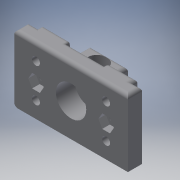
# Autodesk Inventor part: Upper_bearing_support_inside
Saved by Autodesk Inventor 2019.3 (Build 233278000, 278)
## iProperties
Created: 2020-09-08
Part Number: Upper_bearing_support_inside
Material: Generisch
Document SubType Name: Modeling
Designer: Nicolas Frick
Density: 1 g/cm^3
Appearance: Vorgabe
Author: Nicolas Frick
Autodesk Inventor part; units mm, degrees
ref_plane "YZ Plane" through (0, 0, 0) normal (1, 0, 0) x (0, 1, 0)
ref_plane "XZ Plane" through (0, 0, 0) normal (0, 1, 0) x (-1, 0, 0)
ref_plane "XY Plane" through (0, 0, 0) normal (0, 0, 1) x (1, 0, 0)
sketch "Skizze1" plane through (0, 0, 0) normal (0, 0, 1) x (1, 0, 0)
  line L0 (0, 81) -> (-70, 81) construction
  line L1 (-70, 0) -> (-70, 81) construction
  line L2 (-55.2549, 0) -> (-70, 0) construction
  line L3 (-55.2549, 0) -> (-55.2549, 27) construction
  line L4 (-55.2549, 27) -> (-15.0049, 27) construction
  line L5 (-15.0049, 27) -> (-15.0049, 0) construction
  line L6 (0, 0) -> (-15.0049, 0) construction
  line L7 (0, 0) -> (0, 81) construction
  line L8 (-35.1299, 27) -> (-35.1299, 54) construction
  line L9 (-65.1299, 36.5) -> (-5.1299, 36.5)
  line L10 (-5.1299, 36.5) -> (-5.1299, 71.5)
  line L11 (-5.1299, 71.5) -> (-65.1299, 71.5)
  line L12 (-65.1299, 71.5) -> (-65.1299, 36.5)
  line L13 (-65.1299, 36.5) -> (-5.1299, 71.5) construction
  line L14 (-5.1299, 36.5) -> (-65.1299, 71.5) construction
  circle A0 centre (-35.1299, 54) radius 8
  dimension "d0" = 27
  dimension "d1" = 60
  dimension "d2" = 35
  dimension "d3" = 16
  constraints: 14 end point, 3 midpoint, 2 parallel, 1 centre point, 1 coincident, 1 horizontal, 1 perpendicular, 1 vertical
  measures "d0" distance of L8.start L8.end
  measures "d1" distance of L11.end L10.end
  measures "d2" distance of L10.end L9.end
  measures "d3" diameter of A0
extrude "Extrusion1" add sketch "Skizze1" along normal blind 10
sketch "Skizze2" plane through (-65.1299, 71.5, 0) normal (0, 1, 0) x (1, 0, 0)
  line L0 (0, 0) -> (60, 0) construction
  line L1 (60, 0) -> (40, 0) construction
  line L2 (0, 0) -> (0, -10) construction
  line L3 (40, 0) -> (20, 0)
  line L4 (20, 0) -> (20, 10)
  line L5 (20, 10) -> (40, 10)
  line L6 (40, 10) -> (40, 0)
  circle A0 centre (30, 3.7987) radius 3.15
  point P0 (65.1299, 0)
  dimension "d6" = 20
  dimension "d7" = 20
  dimension "d8" = 10
  dimension "d9" = 6.3
  constraints: 10 end point, 2 parallel, 2 perpendicular, 1 centre point, 1 horizontal
  measures "d6" distance of L0.end L1.end
  measures "d7" distance of L4.end L5.end
  measures "d8" distance of L3.end L4.end
  measures "d9" diameter of A0
extrude "Extrusion2" add sketch "Skizze2" against normal up to surface (35 mm away)
sketch "Skizze3" plane through (-65.1299, 36.5, 10) normal (0, -1, 0) x (1, 0, 0)
  circle A0 centre (30, -13.7987) radius 3.15 construction
  line L0 (56.6201, -20) -> (3.6201, -20) construction
  line L1 (42.1201, -18.5) -> (20.1201, -18.5) construction
  line L2 (40, -10) -> (40, -20) construction
  line L3 (20, -20) -> (20, -10) construction
  line L4 (30, -13.7987) -> (24.1, -13.7987) construction
  line L5 (24.1, -13.7987) -> (27.05, -8.6891)
  line L6 (27.05, -8.6891) -> (32.95, -8.6891)
  line L7 (32.95, -8.6891) -> (35.9, -13.7987)
  line L8 (35.9, -13.7987) -> (32.95, -18.9082)
  line L9 (32.95, -18.9082) -> (27.05, -18.9082)
  line L10 (27.05, -18.9082) -> (24.1, -13.7987)
  point P0 (65.1299, -10)
  dimension "d12" = 5.9
  constraints: 14 end point, 1 coincident, 1 horizontal, 13 other
  measures "d12" distance of L4.start L4.end
extrude "Extrusion3" cut sketch "Skizze3" against normal blind 6
sketch "Skizze5" plane through (0, 0, 10) normal (0, 0, 1) x (1, 0, 0)
  circle A0 centre (-16.6299, 63) radius 2.1 projected
  circle A1 centre (-16.6299, 45) radius 2.1 projected
  circle A2 centre (-53.6154, 45) radius 2.1 projected
  circle A3 centre (-53.6154, 63) radius 2.1 projected
  point P0 (0, 0)
extrude "Extrusion4" cut sketch "Skizze5" against normal up to surface (10 mm away)
sketch "Skizze6" plane through (0, 0, 0) normal (0, 0, -1) x (-1, 0, 0)
  circle A0 centre (16.6299, 63) radius 2.1 construction
  circle A1 centre (16.6299, 45) radius 2.1 construction
  circle A2 centre (53.6154, 63) radius 2.1 construction
  circle A3 centre (53.6154, 45) radius 2.1 construction
  line L0 (16.6299, 63) -> (20.7299, 63) construction
  line L1 (16.6299, 45) -> (20.7299, 45) construction
  line L2 (53.6154, 63) -> (49.5154, 63) construction
  line L3 (53.6154, 45) -> (49.5154, 45) construction
  line L4 (20.7299, 63) -> (18.6799, 59.4493)
  line L5 (18.6799, 59.4493) -> (14.5799, 59.4493)
  line L6 (14.5799, 59.4493) -> (12.5299, 63)
  line L7 (12.5299, 63) -> (14.5799, 66.5507)
  line L8 (14.5799, 66.5507) -> (18.6799, 66.5507)
  line L9 (18.6799, 66.5507) -> (20.7299, 63)
  line L10 (49.5154, 63) -> (51.5654, 66.5507)
  line L11 (51.5654, 66.5507) -> (55.6654, 66.5507)
  line L12 (55.6654, 66.5507) -> (57.7154, 63)
  line L13 (57.7154, 63) -> (55.6654, 59.4493)
  line L14 (55.6654, 59.4493) -> (51.5654, 59.4493)
  line L15 (51.5654, 59.4493) -> (49.5154, 63)
  line L16 (49.5154, 45) -> (51.5654, 48.5507)
  line L17 (51.5654, 48.5507) -> (55.6654, 48.5507)
  line L18 (55.6654, 48.5507) -> (57.7154, 45)
  line L19 (57.7154, 45) -> (55.6654, 41.4493)
  line L20 (55.6654, 41.4493) -> (51.5654, 41.4493)
  line L21 (51.5654, 41.4493) -> (49.5154, 45)
  line L22 (20.7299, 45) -> (18.6799, 41.4493)
  line L23 (18.6799, 41.4493) -> (14.5799, 41.4493)
  line L24 (14.5799, 41.4493) -> (12.5299, 45)
  line L25 (12.5299, 45) -> (14.5799, 48.5507)
  line L26 (14.5799, 48.5507) -> (18.6799, 48.5507)
  line L27 (18.6799, 48.5507) -> (20.7299, 45)
  point P0 (0, 0)
  dimension "d17" = 4.1
  dimension "d18" = 4.1
  dimension "d19" = 4.1
  dimension "d20" = 4.1
  constraints: 56 end point, 4 coincident, 4 horizontal, 52 other
  measures "d17" distance of L0.start L0.end
  measures "d18" distance of L1.start L1.end
  measures "d19" distance of L2.start L2.end
  measures "d20" distance of L3.start L3.end
extrude "Extrusion5" cut sketch "Skizze6" against normal blind 4
sketch "Skizze7" plane through (-65.1299, 71.5, 10) normal (0, 1, 0) x (1, 0, 0)
  circle A0 centre (30, 13.7987) radius 3.15 construction
  line L0 (60, 10) -> (40, 10) construction
  line L1 (40, 20) -> (40, 10) construction
  line L2 (20, 20) -> (40, 20) construction
  line L3 (20, 10) -> (20, 20) construction
  line L4 (20, 10) -> (0, 10) construction
  line L5 (0, 10) -> (0, 0) construction
  line L6 (60, 0) -> (0, 0) construction
  line L7 (60, 10) -> (60, 0) construction
  line L8 (-2, 14.15) -> (-2, 9.85) construction
  line L9 (-0.1655, 10.15) -> (-0.1655, 14.15) construction
  line L10 (-2, 14.15) -> (-2, 9.85) construction
  line L11 (-2, 14.15) -> (-2, 9.85) construction
  line L12 (-0.1655, 10.15) -> (-0.1655, 14.15) construction
  line L13 (-2, 9.85) -> (-0.15, 9.85) construction
  line L14 (0, 10) -> (20, 10) projected
  line L15 (0, 10) -> (5, 10)
  line L16 (5, 10) -> (5, 7.5)
  line L17 (5, 7.5) -> (0, 7.5)
  line L18 (0, 7.5) -> (0, 10)
  line L19 (60, 10) -> (55, 10)
  line L20 (55, 10) -> (55, 7.5)
  line L21 (55, 7.5) -> (60, 7.5)
  line L22 (60, 7.5) -> (60, 10)
  point P0 (65.1299, 10)
  dimension "d24" = 5
  dimension "d25" = 2.5
  dimension "d26" = 5
  dimension "d27" = 2.5
  constraints: 18 end point, 4 parallel, 3 horizontal, 2 perpendicular, 1 other
  measures "d24" distance of L16.end L17.end
  measures "d25" distance of L15.end L16.end
  measures "d26" distance of L21.end L20.end
  measures "d27" distance of L20.end L19.end
extrude "Extrusion6" cut sketch "Skizze7" against normal through all
fillet "Rundung2" radius 2 13 edges at (-35.1299, 71.5, 10) (-5.1299, 71.5, 6.25) (-7.6299, 71.5, 2.5) (-17.6299, 71.5, 0) (-25.1299, 71.5, -5) (-10.1299, 71.5, 1.25) (-45.1299, 71.5, -5) (-52.6299, 71.5, 0) (-60.1299, 71.5, 1.25) (-62.6299, 71.5, 2.5) (-65.1299, 71.5, 6.25) (-65.1299, 36.5, 6.25) (-35.1299, 71.5, -10)
fillet "Rundung3" radius 1 1 edges at (-38.2799, 71.5, -3.7987)
sketch "Skizze8" plane through (-63.1299, 71.5, 8) normal (0, 1, 0) x (1, 0, 0)
  line L0 (38, 8) -> (38, 18) projected
  line L1 (18, 18) -> (18, 8) projected
  line L2 (38, 18) -> (18, 18) projected
  line L3 (5, 6) -> (20, 6) projected
  line L4 (38, 18) -> (18, 18)
  line L5 (18, 18) -> (18, 6)
  line L6 (18, 6) -> (38, 6)
  line L7 (38, 6) -> (38, 18)
  point P0 (63.1299, 8)
  constraints: 8 end point, 2 parallel, 1 horizontal, 1 perpendicular, 1 point on line
extrude "Extrusion7" cut sketch "Skizze8" against normal blind 7
sketch "Skizze9" plane through (-63.1299, 64.5, 8) normal (0, 1, 0) x (1, 0, 0)
  circle A0 centre (28, 11.7987) radius 3.15 projected
  point P0 (63.1299, 8)
hole "Bohrung1" at (-35.1299, 64.5, -3.7987) direction (0, -1, 0) diameter 6.3 end through all counterbore diameter 10.3 counterbore depth 10
fillet "Rundung4" radius 2 4 edges at (-35.1299, 71.5, 2) (-25.1299, 64.5, -5) (-35.1299, 64.5, -10) (-45.1299, 64.5, -5)
fillet "Rundung5" radius 1 2 edges at (-26.1299, 64.5, 0) (-44.1299, 64.5, 0)
fillet "Rundung6" radius 1 8 edges at (-45.1299, 64, 0) (-45.1299, 67, 0) (-45.1299, 71.5, 3) (-45.1299, 70.9142, 0.5858) (-25.1299, 70.9142, 0.5858) (-25.1299, 71.5, 3) (-25.1299, 64, 0) (-25.1299, 67, 0)
sketch "Skizze10" plane through (0, 0, 10) normal (0, 0, 1) x (1, 0, 0)
  arc A0 (-65.1299, 38.5) -> (-63.1299, 36.5) centre (-63.1299, 38.5) ccw construction
  line L0 (-63.1299, 36.5) -> (-5.1299, 36.5) construction
  line L1 (-5.1299, 36.5) -> (-5.1299, 69.5) construction
  line L2 (-65.1299, 69.5) -> (-5.1299, 69.5) construction
  line L3 (-65.1299, 69.5) -> (-65.1299, 38.5) construction
  circle A1 centre (-53.6154, 45) radius 2.1 construction
  circle A2 centre (-53.6154, 63) radius 2.1 construction
  circle A3 centre (-16.6299, 45) radius 2.1 construction
  circle A4 centre (-16.6299, 63) radius 2.1 construction
  circle A5 centre (-35.1299, 54) radius 8 construction
  line L4 (-16.6299, 53) -> (-53.6154, 53) construction
  circle A6 centre (-53.6154, 53) radius 2.15
  circle A7 centre (-16.6299, 53) radius 2.15
  point P0 (0, 0)
  dimension "d44" = 4.3
  dimension "d45" = 4.3
  constraints: 2 centre point, 2 coincident, 2 end point, 1 horizontal
  measures "d44" diameter of A6
  measures "d45" diameter of A7
extrude "Extrusion8" cut sketch "Skizze10" against normal through all
sketch "Skizze11" plane through (0, 0, 10) normal (0, 0, 1) x (1, 0, 0)
  circle A0 centre (-16.6299, 53) radius 2.15 construction
  circle A1 centre (-53.6154, 53) radius 2.15 construction
  line L0 (-16.6299, 53) -> (-12.5299, 53) construction
  line L1 (-53.6154, 53) -> (-49.5154, 53) construction
  line L2 (-12.5299, 53) -> (-14.5799, 49.4493)
  line L3 (-14.5799, 49.4493) -> (-18.6799, 49.4493)
  line L4 (-18.6799, 49.4493) -> (-20.7299, 53)
  line L5 (-20.7299, 53) -> (-18.6799, 56.5507)
  line L6 (-18.6799, 56.5507) -> (-14.5799, 56.5507)
  line L7 (-14.5799, 56.5507) -> (-12.5299, 53)
  line L8 (-49.5154, 53) -> (-51.5654, 49.4493)
  line L9 (-51.5654, 49.4493) -> (-55.6654, 49.4493)
  line L10 (-55.6654, 49.4493) -> (-57.7154, 53)
  line L11 (-57.7154, 53) -> (-55.6654, 56.5507)
  line L12 (-55.6654, 56.5507) -> (-51.5654, 56.5507)
  line L13 (-51.5654, 56.5507) -> (-49.5154, 53)
  point P0 (0, 0)
  dimension "d48" = 4.1
  dimension "d49" = 4.1
  constraints: 28 end point, 2 coincident, 2 horizontal, 26 other
  measures "d48" distance of L0.start L0.end
  measures "d49" distance of L1.start L1.end
extrude "Extrusion9" cut sketch "Skizze11" against normal blind 4
